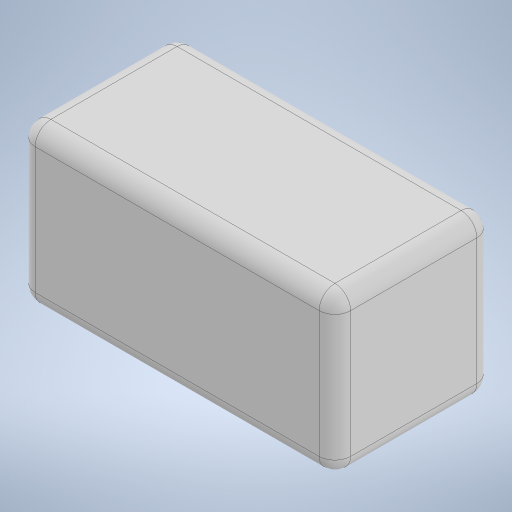
# Autodesk Inventor part: controllerboxv1
Saved by Autodesk Inventor 2024 (Build 280153000, 153)
## iProperties
Created: 2024-04-05
Part Number: controllerboxv1
Material: Generic
Document SubType Name: Modeling
Designer: srika
Density: 1 g/cm^3
Appearance: Default
Author: srika
Autodesk Inventor part; units mm, degrees
ref_plane "YZ Plane" through (0, 0, 0) normal (1, 0, 0) x (0, 1, 0)
ref_plane "XZ Plane" through (0, 0, 0) normal (0, 1, 0) x (-1, 0, 0)
ref_plane "XY Plane" through (0, 0, 0) normal (0, 0, 1) x (1, 0, 0)
sketch "Sketch1" plane through (0, 0, 0) normal (0, 0, 1) x (1, 0, 0)
  line L0 (-50, -25) -> (50, -25)
  line L1 (50, -25) -> (50, 25)
  line L2 (50, 25) -> (-50, 25)
  line L3 (-50, 25) -> (-50, -25)
  line L4 (-50, -25) -> (50, 25) construction
  line L5 (50, -25) -> (-50, 25) construction
  point P0 (0, 0)
  dimension "d0" = 100
  dimension "d1" = 50
  constraints: 12 end point, 2 midpoint, 2 parallel, 1 horizontal, 1 perpendicular
  measures "d0" distance of L1.end L2.end
  measures "d1" distance of L0.end L1.end
extrude "Extrusion1" add sketch "Sketch1" along normal blind 50
fillet "Fillet1" radius 5 12 edges at (50, 0, 50) (50, 0, 0) (-50, 0, 50) (0, 25, 50) (50, 25, 25) (0, 25, 0) (-50, 25, 25) (50, -25, 25) (0, -25, 50) (-50, -25, 25) (-50, 0, 0) (0, -25, 0)
body "Solid1"
